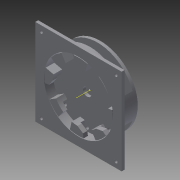
# Autodesk Inventor part: bayonet container 8
Saved by Autodesk Inventor 2015 (Build 190159000, 159)
## iProperties
Created: 2014-09-09
Part Number: bayonet container 8
Material: Generic
Document SubType Name: Modeling
Designer: ericd_000
Density: 1 g/cm^3
Appearance: Default
Author: ericd_000
Autodesk Inventor part; units mm, degrees
ref_plane "YZ Plane" through (0, 0, 0) normal (1, 0, 0) x (0, 1, 0)
ref_plane "XZ Plane" through (0, 0, 0) normal (0, 1, 0) x (-1, 0, 0)
ref_plane "XY Plane" through (0, 0, 0) normal (0, 0, 1) x (1, 0, 0)
sketch "Sketch1" plane through (0, 0, 0) normal (0, 1, 0) x (-1, 0, 0)
  line L0 (75, 75) -> (-75, 75)
  line L1 (-75, 75) -> (-75, -75)
  line L2 (-75, -75) -> (75, -75)
  line L3 (75, -75) -> (75, 75)
  circle A0 centre (0, 0) radius 35
  circle A1 centre (65, 65) radius 2.75
  circle A2 centre (-65, 65) radius 2.75
  circle A3 centre (-65, -65) radius 2.75
  circle A4 centre (65, -65) radius 2.75
  point P0 (75, 0)
  point P1 (0, -75)
  dimension "d0" = 150
  dimension "d1" = 150
  dimension "d2" = 70
  dimension "d3" = 5.5
  dimension "d4" = 10
  dimension "d5" = 10
  dimension "d8" = 360
  constraints: 8 end point, 5 centre point, 2 midpoint, 2 parallel, 1 coincident, 1 horizontal, 1 horizontal alignment, 1 perpendicular, 1 vertical alignment, 9 other
  measures "d0" distance of L2.end L0.start
  measures "d1" distance of L1.end L2.end
  measures "d2" diameter of A0
  measures "d3" diameter of A1
  measures "d4" distance from line of L3 A1.centre
  measures "d5" distance from line of L0 A1.centre
extrude "Extrusion1" add sketch "Sketch1" along normal blind 5
sketch "Sketch2" plane through (0, 0, 0) normal (0, -1, 0) x (1, 0, 0)
  circle A0 centre (0, 0) radius 65
  dimension "d12" = 130
  constraints: 1 centre point, 1 coincident
  measures "d12" diameter of A0
extrude "Extrusion2" cut sketch "Sketch2" against normal blind 10
sketch "Sketch3" plane through (0, 0, 0) normal (0, -1, 0) x (1, 0, 0)
  circle A0 centre (0, 0) radius 65
  circle A1 centre (0, 0) radius 60
  dimension "d15" = 130
  dimension "d16" = 120
  constraints: 2 centre point, 2 coincident
  measures "d15" diameter of A0
  measures "d16" diameter of A1
extrude "Extrusion3" add sketch "Sketch3" against normal blind 20
sketch "Sketch4" plane through (0, 20, 0) normal (0, 1, 0) x (1, 0, 0)
  circle A0 centre (0, 0) radius 60
  point P0 (0, 0)
  dimension "d42" = 120
  constraints: 1 centre point, 1 coincident
  measures "d42" diameter of A0
extrude "Extrusion4" add sketch "Sketch4" against normal blind 5
sketch "Sketch5" plane through (0, 15, 0) normal (0, -1, 0) x (1, 0, 0)
  circle A0 centre (0, 54) radius 3
  point P0 (0, 0)
  dimension "d21" = 6
  dimension "d22" = 54
  constraints: 1 centre point
  measures "d21" diameter of A0
  measures "d22" distance of A0.centre point (0, 0)
extrude "Extrusion5" cut sketch "Sketch5" against normal up to next
pattern_circular "Circular Pattern1" count 8 over 360 about axis through (0, 0, 0) along (0, 1, 0) of "Extrusion5"
sketch "Sketch6" plane through (0, 15, 0) normal (0, -1, 0) x (1, 0, 0)
  circle A0 centre (0, 0) radius 7.5
  point P0 (0, 0)
  dimension "d28" = 15
  constraints: 1 centre point, 1 coincident
  measures "d28" diameter of A0
extrude "Extrusion6" cut sketch "Sketch6" against normal blind 10
sketch "Sketch7" plane through (0, 15, 0) normal (0, -1, 0) x (1, 0, 0)
  circle A0 centre (0, 0) radius 45
  circle A1 centre (0, 0) radius 60 projected
  line L0 (0, 0) -> (-28.7368, 34.6294) construction
  circle A2 centre (-38.1838, 38.1838) radius 3 projected
  line L1 (0, 0) -> (-22.2869, 39.0934) construction
  circle A3 centre (0, 0) radius 59
  line L2 (-22.2869, 39.0934) -> (-29.7159, 50.9702)
  line L3 (-28.7368, 34.6294) -> (-37.6772, 45.403)
  point P0 (-38.3158, 46.1725)
  point P1 (-29.7159, 52.1245)
  dimension "d31" = 15
  dimension "d43" = 120
  dimension "d44" = 118
  dimension "d45" = 14
  constraints: 8 end point, 6 point on circle, 2 centre point, 2 coincident, 1 collinear, 1 point on line
  measures "d31" radial gap between concentric circles of A1 A0
  measures "d43" diameter of A1
  measures "d44" diameter of A3
  measures "d45" radial gap between concentric circles of A3 A0
extrude "Extrusion7" add sketch "Sketch7" along normal blind 15 contours A0 L3 A3 L2 picked at (-33.8469, 42.4787)
sketch "Sketch9" plane through (0, 0, 0) normal (0, -1, 0) x (1, 0, 0)
  circle A0 centre (0, 0) radius 29.9834
  circle A1 centre (0, 0) radius 39.9778
  line L0 (0, 0) -> (-26.8767, 13.2908) construction
  line L1 (-35.8356, 17.721) -> (-26.8767, 13.2908)
  point P0 (0, 0)
  constraints: 4 end point, 2 coincident, 1 collinear, 1 point on line, 6 other
sketch "Sketch10" plane through (-28.7368, 0, 34.6294) normal (-0.769542, 0, -0.6385963) x (-0.6385963, 0, 0.769542)
  line L0 (0, 0) -> (14, 0)
  line L1 (14, 0) -> (14, 7.5)
  line L2 (14, 15) -> (14, 0) projected
  line L3 (0, 15) -> (0, 0) projected
  line L4 (0, 7.5) -> (14, 7.5)
  line L5 (0, 15) -> (14, 15)
  line L6 (-45, -32) -> (-45, 52) projected
  point P0 (-45, 0)
  dimension "d46" = 7.5
  constraints: 8 end point, 2 horizontal, 2 midpoint, 1 parallel
  measures "d46" distance between parallel lines of L0 L4
revolve "Revolution2" add sketch "Sketch10" angle 14 about axis through (0, 0, 0) along (0, -1, 0) contours L3 L4 L1 L0
sketch "Sketch11" plane through (0, 0, 0) normal (0, -1, 0) x (1, 0, 0)
  line L0 (-36.2608, 26.6487) -> (-47.542, 34.9394) projected
  line L1 (-41.9014, 30.794) -> (-30.5426, 33.0477)
  arc A0 (-22.2869, 39.0934) -> (-36.2608, 26.6487) centre (0, 0) ccw projected
  point P0 (0, 0)
  constraints: 2 end point, 1 midpoint, 1 point on circle
extrude "Extrusion8" cut sketch "Sketch11" against normal up to next
pattern_circular "Circular Pattern2" count 8 over 360 about axis through (0, 0, 0) along (0, 1, 0) of "Extrusion7", "Revolution2", "Extrusion8"
sketch "Sketch12" plane through (0, 0, 0) normal (0, -1, 0) x (0.7435557, 0, 0.6686741)
  line L0 (-50.9155, -10.5649) -> (-44.0615, -9.1427)
  line L1 (-50.9155, -10.5649) -> (-57.7695, -11.9871) projected
  arc A0 (-44.9958, -0.612) -> (-44.0615, -9.1427) centre (0, 0) ccw
  arc A1 (-43.9708, 9.5692) -> (-44.9958, -0.612) centre (0, 0) ccw projected
  line L2 (-50.9155, -10.5649) -> (-44.9958, -0.612)
  line L3 (-50.9155, -10.5649) -> (-44.9958, -0.612) projected
  point P0 (0, 0)
  constraints: 4 end point, 2 collinear, 2 point on circle, 1 centre point, 1 concentric
extrude "Extrusion9" add sketch "Sketch12" against normal up to surface (7.5 mm away)
sketch "Sketch13" plane through (0, 20, 0) normal (0, 1, 0) x (1, 0, 0)
  circle A0 centre (0, 0) radius 65
  circle A1 centre (0, 0) radius 61
  dimension "d52" = 4
  dimension "d53" = 130
  constraints: 2 centre point, 2 coincident
  measures "d52" radial gap between concentric circles of A0 A1
  measures "d53" diameter of A0
extrude "Extrusion10" add sketch "Sketch13" along normal blind 13
sketch "Sketch17" plane through (0, 0, 0) normal (0, 0, 1) x (1, 0, 0)
  line L0 (61, 20) -> (-61, 20) projected
  line L1 (61.0173, 20) -> (-61, 20)
  line L2 (-61, 20) -> (-61, 51.3289)
  line L3 (-61, 51.3289) -> (61.0173, 51.3289)
  line L4 (61.0173, 51.3289) -> (61.0173, 20)
  point P0 (0, 0)
  constraints: 8 end point, 2 parallel, 1 horizontal, 1 perpendicular, 1 point on line
extrude "Extrusion13" cut sketch "Sketch17" along normal through all both and the other way through all
sketch "Sketch14" plane through (0, 33, 0) normal (0, 1, 0) x (1, 0, 0)
  circle A0 centre (0, 0) radius 65
  constraints: 1 centre point, 1 coincident
extrude "Extrusion11" add sketch "Sketch14" along normal blind 5
sketch "Sketch18" plane through (0, 20, 0) normal (0, 1, 0) x (1, 0, 0)
  point P0 (0, 0)
sketch "Sketch19" plane through (0, 33, 0) normal (0, -1, 0) x (1, 0, 0)
  circle A0 centre (0, 0) radius 6
  dimension "d63" = 12
  constraints: 1 centre point, 1 coincident
  measures "d63" diameter of A0
extrude "Extrusion14" add sketch "Sketch19" along normal blind 2
body "Solid1"
